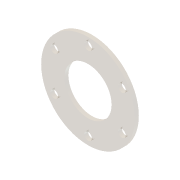
# Autodesk Inventor part: 94 Sprocket Spacer Custom Polycarb
Saved by Autodesk Inventor 2011 (Build 150239000, 239)
## iProperties
Created: 2012-06-05
Part Number: 94 Sprocket Spacer Custom Polycarb
Material: Polycarbonate, Smoke
Document SubType Name: Modeling
Designer: Nemo
Mass: 5.18507 g
Surface Area: 44.8184 cm^2
Volume: 4.32089 cm^3
Density: 1.2 g/cm^3
Author: Nemo
Autodesk Inventor part; units mm, degrees
ref_plane "YZ Plane" through (0, 0, 0) normal (1, 0, 0) x (0, 1, 0)
ref_plane "XZ Plane" through (0, 0, 0) normal (0, 1, 0) x (-1, 0, 0)
ref_plane "XY Plane" through (0, 0, 0) normal (0, 0, 1) x (1, 0, 0)
sketch "Sketch1" plane through (0, 0, 0) normal (0, 0, 1) x (1, 0, 0)
  circle A0 centre (0, 0) radius 28.575
  circle A1 centre (20.6222, 11.9062) radius 2.3818
  circle A2 centre (0, 0) radius 14.351
  circle A3 centre (-20.6222, 11.9062) radius 2.3263
  circle A4 centre (-20.6222, -11.9062) radius 2.3263
  circle A5 centre (0, -23.8125) radius 2.3263
  circle A6 centre (20.6222, -11.9062) radius 2.3263
  circle A7 centre (0, 23.8125) radius 2.3818
  constraints: 8 centre point
extrude "Extrusion1" add sketch "Sketch1" along normal blind 2.3813
body "Solid1"
